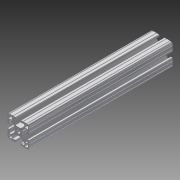
# Autodesk Inventor part: 1515- LITE ALUMINUM PROFILE
Saved by Autodesk Inventor 2014 SP1 (Build 180222100, 222)
## iProperties
Created: 2014-01-21
Part Number: 1515- LITE ALUMINUM PROFILE
Material: Generic
Document SubType Name: Modeling
Designer: Carol
Density: 1 g/cm^3
Appearance: Aluminum - Polished
Author: Carol
Autodesk Inventor part; units mm, degrees
ref_plane "YZ Plane" through (0, 0, 0) normal (1, 0, 0) x (0, 1, 0)
ref_plane "XZ Plane" through (0, 0, 0) normal (0, 1, 0) x (-1, 0, 0)
ref_plane "XY Plane" through (0, 0, 0) normal (0, 0, 1) x (1, 0, 0)
sketch "Sketch1" plane through (0, 0, 0) normal (0, 0, 1) x (1, 0, 0)
  line L0 (6.731, -6.731) -> (-6.731, -6.731)
  line L1 (-6.731, -6.731) -> (-6.731, 2.5767)
  line L2 (-2.5767, 6.731) -> (6.731, 6.731)
  line L3 (6.731, 6.731) -> (6.731, -6.731)
  line L4 (6.731, -6.731) -> (-6.731, 6.731) construction
  line L5 (-6.731, -6.731) -> (6.731, 6.731) construction
  line L6 (0, 0) -> (-31.8372, 31.8372) construction
  line L7 (-5.9892, 8.1445) -> (-10.287, 12.4423)
  line L8 (-8.1445, 5.9892) -> (-12.4423, 10.287)
  line L9 (-10.287, 12.4423) -> (-12.4423, 10.287) construction
  arc A0 (-6.731, 2.5767) -> (-8.1445, 5.9892) centre (-11.557, 2.5767) ccw
  arc A1 (-5.9892, 8.1445) -> (-2.5767, 6.731) centre (-2.5767, 11.557) ccw
  line L10 (-10.5846, 13.1607) -> (-10.5846, 14.9387)
  arc A2 (-10.5846, 13.1607) -> (-10.287, 12.4423) centre (-9.5686, 13.1607) ccw
  arc A3 (-9.3146, 16.2087) -> (-10.5846, 14.9387) centre (-9.3146, 14.9387) ccw
  line L11 (-9.3146, 16.2087) -> (-7.0286, 16.2087)
  line L12 (-7.0286, 16.2087) -> (-7.0286, 15.4467)
  line L13 (-7.0286, 15.4467) -> (-5.7586, 15.4467)
  arc A4 (-5.7586, 15.4467) -> (-4.2346, 16.9707) centre (-5.7586, 16.9707) ccw
  line L14 (-5.7586, 15.4467) -> (-5.7586, 16.9707) construction
  line L15 (-4.2346, 16.9707) -> (-5.7586, 16.9707) construction
  line L16 (-4.2346, 16.9707) -> (-4.2346, 17.9867)
  arc A5 (-4.2346, 17.9867) -> (-5.7586, 19.5107) centre (-5.7586, 17.9867) ccw
  line L17 (-4.2346, 17.9867) -> (-5.7586, 17.9867) construction
  line L18 (-5.7586, 19.5107) -> (-5.7586, 17.9867) construction
  line L19 (-5.7586, 19.5107) -> (-8.0446, 19.5107)
  arc A6 (-9.5686, 19.5107) -> (-8.0446, 19.5107) centre (-8.8066, 19.5107) ccw
  line L20 (-9.5686, 19.5107) -> (-14.3946, 19.5107)
  arc A7 (-15.9186, 19.5107) -> (-14.3946, 19.5107) centre (-15.1566, 19.5107) ccw
  arc A8 (-15.9186, 19.5107) -> (-18.4586, 18.4586) centre (-15.9186, 15.9186) ccw
  arc A9 (-14.9387, 10.5846) -> (-16.2087, 9.3146) centre (-14.9387, 9.3146) ccw
  line L21 (-16.2087, 9.3146) -> (-16.2087, 7.0286)
  line L22 (-16.2087, 7.0286) -> (-15.4467, 7.0286)
  line L23 (-15.4467, 7.0286) -> (-15.4467, 5.7586)
  arc A10 (-16.9707, 4.2346) -> (-15.4467, 5.7586) centre (-16.9707, 5.7586) ccw
  line L24 (-16.9707, 4.2346) -> (-17.9867, 4.2346)
  arc A11 (-19.5107, 5.7586) -> (-17.9867, 4.2346) centre (-17.9867, 5.7586) ccw
  line L25 (-19.5107, 5.7586) -> (-19.5107, 8.0446)
  arc A12 (-19.5107, 8.0446) -> (-19.5107, 9.5686) centre (-19.5107, 8.8066) ccw
  line L26 (-19.5107, 9.5686) -> (-19.5107, 14.3946)
  arc A13 (-19.5107, 14.3946) -> (-19.5107, 15.9186) centre (-19.5107, 15.1566) ccw
  arc A14 (-18.4586, 18.4586) -> (-19.5107, 15.9186) centre (-15.9186, 15.9186) ccw
  line L27 (-13.1607, 10.5846) -> (-14.9387, 10.5846)
  arc A15 (-12.4423, 10.287) -> (-13.1607, 10.5846) centre (-13.1607, 9.5686) ccw
  dimension "d0" = 13.462
  dimension "d1" = 13.462
  dimension "d2" = 1.524
  dimension "d3" = 1.524
  dimension "d4" = 3.556
  dimension "d5" = 4.826
  dimension "d6" = 1.778
  dimension "d7" = 1.016
  dimension "d8" = 1.27
  dimension "d9" = 2.286
  dimension "d10" = 0.762
  dimension "d11" = 1.27
  dimension "d12" = 1.524
  dimension "d13" = 90
  dimension "d14" = 1.016
  dimension "d15" = 1.524
  dimension "d16" = 90
  dimension "d17" = 2.286
  dimension "d19" = 0.762
  dimension "d20" = 4.826
  dimension "d22" = 0.762
  constraints: 57 end point, 32 point on circle, 18 symmetric about line, 16 centre point, 14 tangent, 8 perpendicular, 5 parallel, 3 horizontal alignment, 3 midpoint, 3 point on line, 2 vertical alignment, 1 collinear, 1 equal radius, 1 horizontal, 6 other
  measures "d0" distance of L4.end L2.end
  measures "d1" distance of L0.end L4.end
  measures "d2" distance between parallel lines of L6 L8
  measures "d3" distance between parallel lines of L7 L6
  measures "d4" distance from line of L1 L7.end
  measures "d5" radius of A0
  measures "d6" distance of L10.start L10.end
  measures "d7" radius of A2
  measures "d8" radius of A3
  measures "d9" distance of L11.start L11.end
  measures "d10" distance of L11.end L12.end
  measures "d11" distance of L12.end L13.end
  measures "d12" radius of A4
  measures "d13" angle of L14 L15
  measures "d14" distance of L15.start L16.end
  measures "d15" radius of A5
  measures "d16" angle of L17 L18
  measures "d17" distance of L18.start L19.end
  measures "d19" radius of A6
  measures "d20" distance of L20.start L20.end
  measures "d22" radius of A7
extrude "Extrusion1" add sketch "Sketch1" along normal blind 254
sketch "Sketch4" plane through (0, 0, 254) normal (0, 0, 1) x (1, 0, 0)
  circle A0 centre (0, 0) radius 3.302
  dimension "d31" = 6.604
  constraints: 1 centre point, 1 coincident
  measures "d31" diameter of A0
extrude "Extrusion2" cut sketch "Sketch4" against normal through all
pattern_circular "Circular Pattern2" count 4 over 360 about axis through (0, 0, 254) along (0, 0, -1) of "Extrusion1"
hole "Hole1" at (0, 0, 254) direction (0, 0, -1) diameter 6.604 end through all
sketch "Sketch5" plane through (0, 0, 254) normal (0, 0, 1) x (1, 0, 0)
  circle A0 centre (0, 0) radius 3.302 construction
  line L0 (-14.9387, 10.5846) -> (-13.1607, 10.5846) construction
  line L1 (-12.4423, 10.287) -> (-8.1445, 5.9892) construction
  line L2 (0, 0) -> (-12.2131, 12.2131) construction
  arc A1 (-12.2131, 11.7051) -> (-11.7051, 12.2131) centre (-12.2131, 12.2131) ccw
  line L3 (-11.7051, 12.2131) -> (-11.7051, 16.7851)
  line L4 (-12.2131, 11.7051) -> (-16.7851, 11.7051)
  arc A2 (-17.2931, 12.2131) -> (-16.7851, 11.7051) centre (-16.7851, 12.2131) ccw
  line L5 (-16.7851, 11.7051) -> (-16.7851, 12.2131) construction
  line L6 (-17.2931, 12.2131) -> (-16.7851, 12.2131) construction
  arc A3 (-11.7051, 16.7851) -> (-12.2131, 17.2931) centre (-12.2131, 16.7851) ccw
  line L7 (-11.7051, 16.7851) -> (-12.2131, 16.7851) construction
  line L8 (-12.2131, 17.2931) -> (-12.2131, 16.7851) construction
  line L9 (-12.2131, 17.2931) -> (-14.4991, 17.2931)
  line L10 (-17.2931, 12.2131) -> (-17.2931, 14.4991)
  arc A4 (-14.4991, 17.2931) -> (-17.2931, 14.4991) centre (-14.4991, 14.4991) ccw
  dimension "d46" = 17.272
  dimension "d47" = 0.508
  dimension "d48" = 4.572
  dimension "d49" = 4.572
  dimension "d50" = 0.508
  dimension "d51" = 90
  dimension "d52" = 0.508
  dimension "d53" = 90
  dimension "d54" = 2.286
  dimension "d55" = 2.286
  constraints: 18 end point, 8 point on circle, 7 tangent, 4 centre point, 3 perpendicular, 1 coincident, 1 horizontal alignment, 1 parallel, 1 vertical alignment
  measures "d46" distance of L2.start L2.end
  measures "d47" radius of A1
  measures "d48" distance of L3.start L3.end
  measures "d49" distance of L4.start L4.end
  measures "d50" radius of A2
  measures "d51" angle of L6 L5
  measures "d52" radius of A3
  measures "d53" angle of L7 L8
  measures "d54" distance of L8.start L9.end
  measures "d55" distance of L6.start L10.end
extrude "Extrusion3" cut sketch "Sketch5" against normal through all
pattern_circular "Circular Pattern3" count 4 over 360 about axis through (0, 0, -5.9256) along (0, 0, 1) of "Extrusion3"
body "Solid1"
